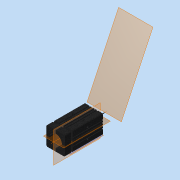
# Autodesk Inventor part: 00_Laser_532nm_200mw
Saved by Autodesk Inventor 2019.4 (Build 234330000, 330)
## iProperties
Created: 2019-08-28
Part Number: 00_Laser_532nm_200mw
Material: Generic
Document SubType Name: Modeling
Designer: diederichbenedict
Density: 1 g/cm^3
Appearance: Black Cast
Mass: 47.2416 g
Surface Area: 127.634 cm^2
Volume: 47.2416 cm^3
Author: diederichbenedict
Autodesk Inventor part; units mm, degrees
ref_plane "YZ Plane" through (0, 0, 0) normal (1, 0, 0) x (0, 1, 0)
ref_plane "XZ Plane" through (0, 0, 0) normal (0, 1, 0) x (-1, 0, 0)
ref_plane "XY Plane" through (0, 0, 0) normal (0, 0, 1) x (1, 0, 0)
sketch "Sketch1" plane through (0, 0, 0) normal (0, 0, 1) x (1, 0, 0)
  line L0 (326.6896, 158.5405) -> (300.7896, 158.5405)
  line L1 (298.7896, 156.5405) -> (298.7896, 130.6405)
  line L2 (300.7896, 128.6405) -> (326.6896, 128.6405)
  line L3 (328.6896, 130.6405) -> (328.6896, 156.5405)
  arc A0 (328.6896, 156.5405) -> (326.6896, 158.5405) centre (326.6896, 156.5405) ccw
  arc A1 (298.7896, 130.6405) -> (300.7896, 128.6405) centre (300.7896, 130.6405) ccw
  arc A2 (300.7896, 158.5405) -> (298.7896, 156.5405) centre (300.7896, 156.5405) ccw
  arc A3 (326.6896, 128.6405) -> (328.6896, 130.6405) centre (326.6896, 130.6405) ccw
  point P0 (0, 0)
  point P1 (298.7896, 128.6405)
  point P2 (298.7896, 158.5405)
  point P3 (328.6896, 128.6405)
  dimension "d0" = 29.9
  dimension "d1" = 29.9
  dimension "d2" = 2
  constraints: 8 end point, 8 point on circle, 8 tangent, 6 point on line, 4 centre point, 3 equal radius, 2 parallel, 1 horizontal, 1 perpendicular
  measures "d0" distance of point (328.69, 128.64) point (298.79, 128.64)
  measures "d1" distance of point (298.79, 128.64) point (298.79, 158.54)
  measures "d2" radius of A0
extrude "Extrusion1" add sketch "Sketch1" along normal blind 48.23
sketch "Sketch2" plane through (0, 0, 0) normal (0, 0, -1) x (-1, 0, 0)
  line L0 (-328.6896, 156.5405) -> (-328.6896, 130.6405) projected
  arc A0 (-328.6896, 130.6405) -> (-326.6896, 128.6405) centre (-326.6896, 130.6405) ccw projected
  line L1 (-326.6896, 128.6405) -> (-300.7896, 128.6405) projected
  arc A1 (-300.7896, 128.6405) -> (-298.7896, 130.6405) centre (-300.7896, 130.6405) ccw projected
  line L2 (-298.7896, 130.6405) -> (-298.7896, 156.5405) projected
  arc A2 (-298.7896, 156.5405) -> (-300.7896, 158.5405) centre (-300.7896, 156.5405) ccw projected
  line L3 (-300.7896, 158.5405) -> (-326.6896, 158.5405) projected
  arc A3 (-326.6896, 158.5405) -> (-328.6896, 156.5405) centre (-326.6896, 156.5405) ccw projected
  circle A4 centre (-313.7396, 143.5905) radius 6.35
  point P0 (0, 0)
  dimension "d5" = 12.7
  constraints: 1 centre point
  measures "d5" diameter of A4
extrude "Extrusion2" add sketch "Sketch2" along normal blind 7 contours A4
sketch "Sketch3" plane through (328.6896, 130.6405, 0) normal (1, 0, 0) x (0, 0, -1)
  line L0 (0, 25.9) -> (0, 0) projected
  line L1 (0, 25.9) -> (-48.23, 25.9) projected
  line L2 (-48.23, 0) -> (-48.23, 25.9) projected
  line L3 (0, 0) -> (-48.23, 0) projected
  line L4 (7, 6.6) -> (7, 19.3) projected
  line L5 (7, 12.95) -> (-48.23, 12.95)
  line L6 (-48.23, 0) -> (-48.23, 25.9) projected
  line L7 (0, 25.9) -> (0, 0) projected
  line L8 (-48.23, 13.95) -> (0, 13.95)
  line L9 (0, 13.95) -> (0, 15.95)
  line L10 (0, 15.95) -> (-48.23, 15.95)
  line L11 (-48.23, 15.95) -> (-48.23, 13.95)
  line L12 (-48.23, 17.95) -> (0, 17.95)
  line L13 (0, 17.95) -> (0, 19.95)
  line L14 (0, 19.95) -> (-48.23, 19.95)
  line L15 (-48.23, 19.95) -> (-48.23, 17.95)
  line L16 (-48.23, 11.95) -> (0, 11.95)
  line L17 (0, 11.95) -> (0, 9.95)
  line L18 (0, 9.95) -> (-48.23, 9.95)
  line L19 (-48.23, 9.95) -> (-48.23, 11.95)
  line L20 (-48.23, 7.95) -> (0, 7.95)
  line L21 (0, 7.95) -> (0, 5.95)
  line L22 (0, 5.95) -> (-48.23, 5.95)
  line L23 (-48.23, 5.95) -> (-48.23, 7.95)
  point P0 (0, -130.6405)
  point P1 (0, 6.95)
  point P2 (0, 10.95)
  dimension "d8" = 2
  dimension "d9" = 1
  dimension "d10" = 2
  dimension "d11" = 2
  dimension "d12" = 2
  dimension "d13" = 1
  dimension "d14" = 2
  dimension "d15" = 2
  constraints: 34 end point, 8 parallel, 8 point on line, 4 horizontal, 4 midpoint, 4 perpendicular
  measures "d8" distance of L9.end L8.end
  measures "d9" distance between parallel lines of L5 L8
  measures "d10" distance of L13.end L12.end
  measures "d11" distance of L16.end L17.end
  measures "d12" distance of L20.end L21.end
  measures "d13" distance between parallel lines of L16 L5
  measures "d14" distance between parallel lines of L20 L18
  measures "d15" distance between parallel lines of L10 L12
extrude "Extrusion3" cut sketch "Sketch3" against normal blind 1 contours L0 L12 L2 L14 | L0 L8 L2 L10 | L0 L18 L2 L16 | L0 L22 L2 L20
pattern_circular "Circular Pattern1" count 4 over 360 about axis through (313.7396, 143.5905, 0) along (0, 0, -1) of "Extrusion3"
sketch "Sketch4" plane through (328.6896, 130.6405, 48.23) normal (1, 0, 0) x (0, 0, -1)
  line L0 (0, 19.95) -> (48.23, 19.95) projected
  line L1 (48.23, 25.9) -> (48.23, 19.95) projected
  line L2 (48.23, 25.9) -> (0, 25.9) projected
  line L3 (0, 19.95) -> (0, 25.9) projected
  line L4 (48.23, 5.95) -> (0, 5.95) projected
  line L5 (0, 0) -> (0, 5.95) projected
  line L6 (48.23, 0) -> (0, 0) projected
  line L7 (48.23, 5.95) -> (48.23, 0) projected
  line L8 (48.23, 27.9) -> (0, 27.9) projected
  line L9 (48.23, -2) -> (0, -2) projected
  point P0 (48.23, -130.6405)
  point P1 (23.73, 21.1)
  point P2 (23.73, 4.8)
  dimension "d21" = 24.5
  dimension "d22" = 24.5
  dimension "d23" = 6.8
  dimension "d24" = 6.8
  measures "d21" distance from line of point (23.73, 21.1) L1
  measures "d22" distance from line of point (23.73, 4.8) L7
  measures "d23" distance from line of point (23.73, 21.1) L8
  measures "d24" distance from line of L9 point (23.73, 4.8)
hole "Hole1" at (328.6896, 135.4405, 24.5) at (328.6896, 151.7405, 24.5) direction (-1, 0, 0) diameter 2.8 depth 12 tip angle 118
sketch "Sketch5" plane through (0, 0, 48.23) normal (0, 0, 1) x (1, 0, 0)
  circle A0 centre (313.7396, 143.5905) radius 6.35 projected
  line L0 (302.7396, 132.5905) -> (324.7396, 132.5905)
  line L1 (324.7396, 132.5905) -> (324.7396, 154.5905)
  line L2 (324.7396, 154.5905) -> (302.7396, 154.5905)
  line L3 (302.7396, 154.5905) -> (302.7396, 132.5905)
  line L4 (302.7396, 132.5905) -> (324.7396, 154.5905) construction
  line L5 (324.7396, 132.5905) -> (302.7396, 154.5905) construction
  circle A1 centre (324.7396, 154.5905) radius 1
  circle A2 centre (324.7396, 132.5905) radius 1
  circle A3 centre (302.7396, 132.5905) radius 1
  circle A4 centre (302.7396, 154.5905) radius 1
  point P0 (0, 0)
  dimension "d32" = 22
  dimension "d33" = 22
  dimension "d34" = 2
  dimension "d35" = 2
  dimension "d36" = 2
  dimension "d37" = 2
  constraints: 12 end point, 4 centre point, 4 coincident, 2 midpoint, 2 parallel, 1 horizontal, 1 perpendicular
  measures "d32" distance of L2.end L1.end
  measures "d33" distance of L1.end L0.end
  measures "d34" diameter of A1
  measures "d35" diameter of A2
  measures "d36" diameter of A3
  measures "d37" diameter of A4
extrude "Extrusion4" add sketch "Sketch5" along normal blind 3 contours L3 A3 L0 | L0 A3 L3 | A2 L1 L0 | L0 L1 A2 | A4 L2 L3 | L3 L2 A4 | A1 L2 L1 | L1 L2 A1
sketch "Sketch6" plane through (324.7396, 154.5905, 51.23) normal (0, 0, 1) x (1, 0, 0)
  circle A0 centre (-22, 0) radius 1 construction
  circle A1 centre (0, -22) radius 1 construction
  circle A2 centre (0, 0) radius 1 construction
  circle A3 centre (-22, -22) radius 1 construction
  line L0 (-12, 3.95) -> (-12, 2.95) construction
  line L1 (-12, 2.95) -> (-14, 2.95) construction
  line L2 (-14, 2.95) -> (-14, 3.95) construction
  line L3 (-14, 3.95) -> (-16, 3.95) construction
  line L4 (-16, 3.95) -> (-16, 2.95) construction
  line L5 (-16, 2.95) -> (-18, 2.95) construction
  line L6 (-18, 2.95) -> (-18, 3.95) construction
  line L7 (-18, 3.95) -> (-23.95, 3.95) construction
  arc A4 (-23.95, 3.95) -> (-25.95, 1.95) centre (-23.95, 1.95) ccw construction
  line L8 (-25.95, 1.95) -> (-25.95, -4) construction
  line L9 (-25.95, -4) -> (-24.95, -4) construction
  line L10 (-24.95, -4) -> (-24.95, -6) construction
  line L11 (-24.95, -6) -> (-25.95, -6) construction
  line L12 (-25.95, -6) -> (-25.95, -8) construction
  line L13 (-25.95, -8) -> (-24.95, -8) construction
  line L14 (-24.95, -8) -> (-24.95, -10) construction
  line L15 (-24.95, -10) -> (-25.95, -10) construction
  line L16 (-25.95, -10) -> (-25.95, -12) construction
  line L17 (-25.95, -12) -> (-24.95, -12) construction
  line L18 (-24.95, -12) -> (-24.95, -14) construction
  line L19 (-24.95, -14) -> (-25.95, -14) construction
  line L20 (-25.95, -14) -> (-25.95, -16) construction
  line L21 (-25.95, -16) -> (-24.95, -16) construction
  line L22 (-24.95, -16) -> (-24.95, -18) construction
  line L23 (-24.95, -18) -> (-25.95, -18) construction
  line L24 (-25.95, -18) -> (-25.95, -23.95) construction
  arc A5 (-25.95, -23.95) -> (-23.95, -25.95) centre (-23.95, -23.95) ccw construction
  line L25 (-23.95, -25.95) -> (-18, -25.95) construction
  line L26 (-18, -25.95) -> (-18, -24.95) construction
  line L27 (-18, -24.95) -> (-16, -24.95) construction
  line L28 (-16, -24.95) -> (-16, -25.95) construction
  line L29 (-16, -25.95) -> (-14, -25.95) construction
  line L30 (-14, -25.95) -> (-14, -24.95) construction
  line L31 (-14, -24.95) -> (-12, -24.95) construction
  line L32 (-12, -24.95) -> (-12, -25.95) construction
  line L33 (-12, -25.95) -> (-10, -25.95) construction
  line L34 (-10, -25.95) -> (-10, -24.95) construction
  line L35 (-10, -24.95) -> (-8, -24.95) construction
  line L36 (-8, -24.95) -> (-8, -25.95) construction
  line L37 (-8, -25.95) -> (-6, -25.95) construction
  line L38 (-6, -25.95) -> (-6, -24.95) construction
  line L39 (-6, -24.95) -> (-4, -24.95) construction
  line L40 (-4, -24.95) -> (-4, -25.95) construction
  line L41 (-4, -25.95) -> (1.95, -25.95) construction
  arc A6 (1.95, -25.95) -> (3.95, -23.95) centre (1.95, -23.95) ccw construction
  line L42 (3.95, -23.95) -> (3.95, -18) construction
  line L43 (3.95, -18) -> (2.95, -18) construction
  line L44 (2.95, -18) -> (2.95, -16) construction
  line L45 (2.95, -16) -> (3.95, -16) construction
  line L46 (3.95, -16) -> (3.95, -14) construction
  line L47 (3.95, -14) -> (2.95, -14) construction
  line L48 (2.95, -14) -> (2.95, -12) construction
  line L49 (2.95, -12) -> (3.95, -12) construction
  line L50 (3.95, -12) -> (3.95, -10) construction
  line L51 (3.95, -10) -> (2.95, -10) construction
  line L52 (2.95, -10) -> (2.95, -8) construction
  line L53 (2.95, -8) -> (3.95, -8) construction
  line L54 (3.95, -8) -> (3.95, -6) construction
  line L55 (3.95, -6) -> (2.95, -6) construction
  line L56 (2.95, -6) -> (2.95, -4) construction
  line L57 (2.95, -4) -> (3.95, -4) construction
  line L58 (3.95, -4) -> (3.95, 1.95) construction
  arc A7 (3.95, 1.95) -> (1.95, 3.95) centre (1.95, 1.95) ccw construction
  line L59 (1.95, 3.95) -> (-4, 3.95) construction
  line L60 (-4, 3.95) -> (-4, 2.95) construction
  line L61 (-4, 2.95) -> (-6, 2.95) construction
  line L62 (-6, 2.95) -> (-6, 3.95) construction
  line L63 (-6, 3.95) -> (-8, 3.95) construction
  line L64 (-8, 3.95) -> (-8, 2.95) construction
  line L65 (-8, 2.95) -> (-10, 2.95) construction
  line L66 (-10, 2.95) -> (-10, 3.95) construction
  line L67 (-10, 3.95) -> (-12, 3.95) construction
  line L68 (-23.95, 3.95) -> (1.95, 3.95)
  line L69 (3.95, 1.95) -> (3.95, -23.95)
  line L70 (1.95, -25.95) -> (-23.95, -25.95)
  line L71 (-25.95, -23.95) -> (-25.95, 1.95)
  arc A8 (-23.95, 3.95) -> (-25.95, 1.95) centre (-23.95, 1.95) ccw
  arc A9 (3.95, 1.95) -> (1.95, 3.95) centre (1.95, 1.95) ccw
  arc A10 (1.95, -25.95) -> (3.95, -23.95) centre (1.95, -23.95) ccw
  arc A11 (-25.95, -23.95) -> (-23.95, -25.95) centre (-23.95, -23.95) ccw
  circle A12 centre (-11, -11) radius 9.9557
  point P0 (-324.7396, -154.5905)
  dimension "d40" = 2
  constraints: 8 end point, 8 point on circle, 8 tangent, 5 centre point, 3 equal radius, 2 parallel, 1 horizontal, 1 perpendicular
  measures "d40" radius of A8
extrude "Extrusion5" add sketch "Sketch6" along normal blind 9.4
ref_plane "Work Plane1" through (326.6896, 126.1405, 0) normal (0, -1, 0) x (1, 0, 0)
ref_plane "Work Plane2" through (326.6896, 143.5905, 48.23) normal (0, 1, 0) x (1, 0, 0)
ref_plane "Work Plane3" through (313.7396, 156.5405, 48.23) normal (1, 0, 0) x (0, 0, -1)
sketch "Sketch8" plane through (313.7396, 143.5905, -7) normal (0, 0, -1) x (-1, 0, 0)
  circle A0 centre (0, 0) radius 6.35 projected
  circle A1 centre (0, 0) radius 6.35 projected
  circle A2 centre (0, 0) radius 0.5
  point P0 (313.7396, -143.5905)
  dimension "d46" = 1
  constraints: 1 centre point, 1 coincident
  measures "d46" diameter of A2
extrude "Extrusion7" add sketch "Sketch8" along normal blind 10 contours A2
pattern_circular "Circular Pattern2" count 4 over 360 about axis through (313.7396, 143.5905, 0) along (0, 0, -1) of "Hole1"
ref_plane "Work Plane4" through (280.0146, 184.3442, -59.8557) normal (0, 0.4305, 0.9026) x (0, 0.9026, -0.4305)
sketch "Sketch9" plane through (280.0146, 184.3442, -59.8557) normal (0, 0.4305, 0.9026) x (0, 0.9026, -0.4305)
  arc A0 (-30.7028, -21.1512) -> (-30.7028, -46.2569) centre (-20.7819, -33.704) ccw projected
  arc A1 (-10.8609, -46.2569) -> (-10.8609, -21.1512) centre (-20.7819, -33.704) ccw projected
  circle A2 centre (-20.7819, -33.704) radius 0.521
  line L0 (-59.5386, -34.225) -> (-55.2335, -34.225) projected
  line L1 (0.271, -16.8756) -> (5.1683, -16.8756)
  line L2 (5.1683, -16.8756) -> (5.1683, -18.1812)
  line L3 (5.1683, -18.1812) -> (0.271, -18.1812)
  line L4 (0.271, -18.1812) -> (0.271, -16.8756)
  point P0 (-192.1549, 280.0146)
  constraints: 8 end point, 2 parallel, 1 centre point, 1 coincident, 1 horizontal, 1 perpendicular, 1 tangent
extrude "Extrusion8" cut sketch "Sketch9" along normal blind 10
body "Solid1"
